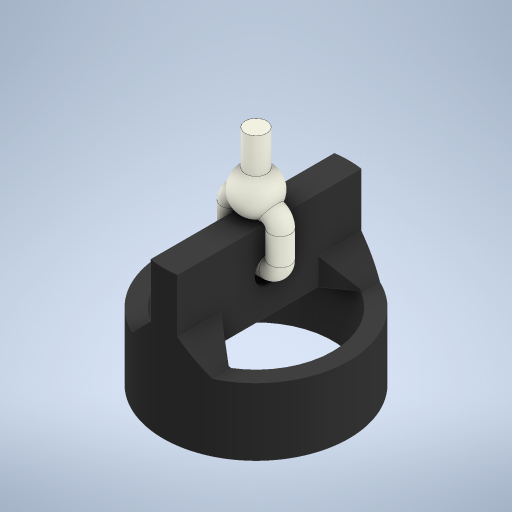
# Autodesk Inventor part: dummy_terminal_end_4.1mm_5.7mm_addon_with_string
Saved by Autodesk Inventor 2024.3 (Build 283343000, 343)
## iProperties
Created: 2024-04-25
Part Number: dummy_terminal_end_4.1mm_5.7mm_addon_with_string
Material: 일반
Document SubType Name: Modeling
Designer: Gihyeok Na
Density: 1 g/cm^3
Appearance: 기본값
Author: Gihyeok Na
Autodesk Inventor part; units mm, degrees
ref_plane "YZ Plane" through (0, 0, 0) normal (1, 0, 0) x (0, 1, 0)
ref_plane "XZ Plane" through (0, 0, 0) normal (0, 1, 0) x (-1, 0, 0)
sketch "스케치1" plane through (0, 0, 0) normal (0, 1, 0) x (-1, 0, 0)
  circle A0 centre (0, 0) radius 2.85
  circle A1 centre (0, 0) radius 3.45
  dimension "d0" = 5.7
  dimension "d1" = 6.9
  constraints: 2 centre point, 2 coincident
  measures "d0" diameter of A0
  measures "d1" diameter of A1
extrude "돌출1" add sketch "스케치1" along normal blind 2.5
sketch "스케치2" plane through (0, 2.5, 0) normal (0, 1, 0) x (1, 0, 0)
  circle A0 centre (0, 0) radius 3.45 projected
  circle A1 centre (0, 0) radius 3.45 projected
  line L0 (0.5, 3.4136) -> (-0.5, 3.4136)
  line L1 (-0.5, 3.4136) -> (-0.5, -3.4136)
  line L2 (-0.5, -3.4136) -> (0.5, -3.4136)
  line L3 (0.5, -3.4136) -> (0.5, 3.4136)
  line L4 (0.5, 3.4136) -> (-0.5, -3.4136) construction
  line L5 (-0.5, 3.4136) -> (0.5, -3.4136) construction
  point P0 (-0.5, -3.4136)
  point P1 (0.5, -3.4136)
  point P2 (0.5, 3.4136)
  point P3 (-0.5, 3.4136)
  dimension "d4" = 1
  constraints: 12 end point, 2 midpoint, 2 parallel, 1 horizontal, 1 perpendicular, 1 point on circle
  measures "d4" distance of L2.end L1.end
extrude "돌출2" add sketch "스케치2" along normal blind 3 contours L0 A0 | L3 L2 L1 L0 | A0 L2
chamfer "모따기1" distance 1 angle 45 4 edges at (0.5, 2.5, 3.1097) (0.5, 2.5, -3.1097) (-0.5, 2.5, -3.1097) (-0.5, 2.5, 3.1097)
chamfer "모따기2" distance 1 angle 45 4 edges at (-0.5, 3, -2.8058) (-0.5, 3, 2.8058) (0.5, 3, 2.8058) (0.5, 3, -2.8058)
sketch "스케치5" plane through (0.5, 5.5, 3.4136) normal (1, 0, 0) x (0, 0, -1)
  line L0 (5.2194, -2) -> (5.2194, -3) projected
  line L1 (6.8272, -2) -> (5.2194, -2) projected
  line L2 (6.8272, -2) -> (6.8272, 0) projected
  line L3 (0, 0) -> (6.8272, 0) projected
  line L4 (0, -2) -> (0, 0) projected
  line L5 (1.6078, -2) -> (0, -2) projected
  line L6 (1.6078, -3) -> (1.6078, -2) projected
  line L7 (1.6078, -3) -> (5.2194, -3) projected
  circle A0 centre (3.363, -1.5) radius 0.5
  line L8 (6.5204, -3) -> (0.3067, -3) projected
  point P0 (3.4136, -5.5)
  dimension "d15" = 1
  dimension "d16" = 1.5
  constraints: 1 centre point
  measures "d15" diameter of A0
  measures "d16" distance from line of L7 A0.centre
extrude "돌출4" cut sketch "스케치5" against normal blind 3 contours A0
sketch "Sketch6" plane through (0, 0, 0) normal (0, 0, 1) x (1, 0, 0)
  line L0 (-0.5, 4.1) -> (0.5, 4.1)
  line L1 (0.9, 4.5) -> (0.9, 5.5)
  line L2 (0.5, 5.9) -> (-0.5, 5.9)
  line L3 (-0.9, 5.5) -> (-0.9, 4.5)
  line L4 (-0.5, 3.5) -> (-1.5, 2.5) projected
  line L5 (-0.5, 3.5) -> (-0.5, 5.5) projected
  line L6 (0.5, 5.5) -> (-0.5, 5.5) projected
  line L7 (0.5, 3.5) -> (0.5, 5.5) projected
  line L8 (1.5, 2.5) -> (0.5, 3.5) projected
  line L9 (1.5, 2.5) -> (1.5, 2.5) projected
  line L10 (0.5, 3.5) -> (1.5, 2.5) projected
  line L11 (0.5, 3.5) -> (0.5, 5.5) projected
  line L12 (-0.5, 5.5) -> (0.5, 5.5) projected
  line L13 (-0.5, 3.5) -> (-0.5, 5.5) projected
  line L14 (-1.5, 2.5) -> (-0.5, 3.5) projected
  line L15 (-1.5, 2.5) -> (-1.5, 2.5) projected
  line L16 (3.45, 0) -> (-3.45, 0) projected
  arc A0 (0.9, 5.5) -> (0.5, 5.9) centre (0.5, 5.5) ccw
  line L17 (0.5, 3.5) -> (0.5, 5.5) projected
  arc A1 (0.5, 4.1) -> (0.9, 4.5) centre (0.5, 4.5) ccw
  arc A2 (-0.9, 4.5) -> (-0.5, 4.1) centre (-0.5, 4.5) ccw
  arc A3 (-0.5, 5.9) -> (-0.9, 5.5) centre (-0.5, 5.5) ccw
  point P0 (0, 0)
  point P1 (0, 5)
  dimension "d21" = 0.4
  constraints: 8 end point, 8 point on circle, 4 centre point, 3 point on line, 2 coincident, 2 midpoint, 2 parallel, 1 horizontal, 1 perpendicular
  measures "d21" distance between parallel lines of L2 L6
sketch "Sketch7" plane through (0, 0, 0) normal (1, 0, 0) x (0, 1, 0)
  line L0 (5.9, 0) -> (5.5, 0) projected
  circle A0 centre (5.9, 0) radius 0.39
  point P0 (0, 0)
  dimension "d22" = 0.78
  constraints: 1 centre point, 1 coincident
  measures "d22" diameter of A0
sweep "Sweep1" add profiles "Sketch7" path "Sketch6" path curves L2 A3 L3 A2 L0 A1 L1 A0
ref_plane "Work Plane1" through (0, 6.3, 0) normal (0, 1, 0) x (1, 0, 0)
sketch "Sketch8" plane through (0, 6.3, 0) normal (0, 1, 0) x (1, 0, 0)
  circle A0 centre (0, 0) radius 0.8
  line L0 (0.8, 0) -> (-0.8, 0)
  dimension "d26" = 1.6
  constraints: 2 end point, 2 point on circle, 1 centre point, 1 coincident, 1 horizontal
  measures "d26" diameter of A0
revolve "Revolution1" add sketch "Sketch8" angle 360 about axis through (0.8, 6.3, 0) along (-1, 0, 0) picked at (0.1996, 0.1768) contours L0 A0
sketch "Sketch9" plane through (0, 6.3, 0) normal (0, 1, 0) x (1, 0, 0)
  circle A0 centre (0, 0) radius 0.4
  dimension "d28" = 0.8
  constraints: 1 centre point, 1 coincident
  measures "d28" diameter of A0
extrude "Extrusion5" add sketch "Sketch9" along normal blind 2
